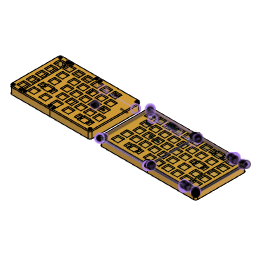
my-keyboard (Autodesk Fusion 360 design; units mm, degrees)
Autodesk Fusion 360 part; units mm, degrees
(part 1 of 2)
sketch "스케치1" plane through (0, 0, 0) normal (0, 0, 1) x (1, 0, 0)
  line L0 (0, 0) -> (143.11, 0)
  line L1 (143.11, 0) -> (143.11, 105.25)
  line L2 (143.11, 105.25) -> (0, 105.25)
  line L3 (0, 105.25) -> (0, 0)
  line L4 (0, 5) -> (143.11, 5) construction
  line L5 (0, 24.05) -> (143.11, 24.05) construction
  line L6 (0, 43.1) -> (143.11, 43.1) construction
  line L7 (0, 62.15) -> (143.11, 62.15) construction
  line L8 (0, 81.2) -> (143.11, 81.2) construction
  line L9 (2.525, 97.725) -> (16.525, 97.725)
  line L10 (16.525, 97.725) -> (16.525, 83.725)
  line L11 (16.525, 83.725) -> (2.525, 83.725)
  line L12 (2.525, 83.725) -> (2.525, 97.725)
  line L13 (7.2875, 64.675) -> (7.2875, 78.675)
  line L14 (7.2875, 78.675) -> (21.2875, 78.675)
  line L15 (21.2875, 78.675) -> (21.2875, 64.675)
  line L16 (21.2875, 64.675) -> (7.2875, 64.675)
  line L17 (21.575, 97.725) -> (35.575, 97.725)
  line L18 (21.575, 83.725) -> (21.575, 97.725)
  line L19 (35.575, 97.725) -> (35.575, 83.725)
  line L20 (35.575, 83.725) -> (21.575, 83.725)
  line L21 (40.625, 97.725) -> (54.625, 97.725)
  line L22 (40.625, 83.725) -> (40.625, 97.725)
  line L23 (54.625, 97.725) -> (54.625, 83.725)
  line L24 (54.625, 83.725) -> (40.625, 83.725)
  line L25 (59.675, 97.725) -> (73.675, 97.725)
  line L26 (59.675, 83.725) -> (59.675, 97.725)
  line L27 (73.675, 97.725) -> (73.675, 83.725)
  line L28 (73.675, 83.725) -> (59.675, 83.725)
  line L29 (78.725, 97.725) -> (92.725, 97.725)
  line L30 (78.725, 83.725) -> (78.725, 97.725)
  line L31 (92.725, 97.725) -> (92.725, 83.725)
  line L32 (92.725, 83.725) -> (78.725, 83.725)
  line L33 (97.775, 97.725) -> (111.775, 97.725)
  line L34 (97.775, 83.725) -> (97.775, 97.725)
  line L35 (111.775, 97.725) -> (111.775, 83.725)
  line L36 (111.775, 83.725) -> (97.775, 83.725)
  line L37 (31.1, 64.675) -> (31.1, 78.675)
  line L38 (31.1, 78.675) -> (45.1, 78.675)
  line L39 (45.1, 78.675) -> (45.1, 64.675)
  line L40 (45.1, 64.675) -> (31.1, 64.675)
  line L41 (64.15, 64.675) -> (50.15, 64.675)
  line L42 (64.15, 78.675) -> (64.15, 64.675)
  line L43 (50.15, 78.675) -> (64.15, 78.675)
  line L44 (50.15, 64.675) -> (50.15, 78.675)
  line L45 (83.2, 64.675) -> (69.2, 64.675)
  line L46 (83.2, 78.675) -> (83.2, 64.675)
  line L47 (69.2, 78.675) -> (83.2, 78.675)
  line L48 (69.2, 64.675) -> (69.2, 78.675)
  line L49 (102.25, 64.675) -> (88.25, 64.675)
  line L50 (102.25, 78.675) -> (102.25, 64.675)
  line L51 (88.25, 78.675) -> (102.25, 78.675)
  line L52 (88.25, 64.675) -> (88.25, 78.675)
  line L53 (121.3, 64.675) -> (107.3, 64.675)
  line L54 (121.3, 78.675) -> (121.3, 64.675)
  line L55 (107.3, 78.675) -> (121.3, 78.675)
  line L56 (107.3, 64.675) -> (107.3, 78.675)
  line L57 (23.66, 59.625) -> (23.66, 45.625)
  line L58 (9.66, 59.625) -> (23.66, 59.625)
  line L59 (9.66, 45.625) -> (9.66, 59.625)
  line L60 (23.66, 45.625) -> (9.66, 45.625)
  line L61 (35.845, 59.625) -> (49.845, 59.625)
  line L62 (35.845, 45.625) -> (35.845, 59.625)
  line L63 (49.845, 59.625) -> (49.845, 45.625)
  line L64 (49.845, 45.625) -> (35.845, 45.625)
  line L65 (54.895, 59.625) -> (68.895, 59.625)
  line L66 (54.895, 45.625) -> (54.895, 59.625)
  line L67 (68.895, 45.625) -> (54.895, 45.625)
  line L68 (68.895, 59.625) -> (68.895, 45.625)
  line L69 (73.945, 59.625) -> (87.945, 59.625)
  line L70 (73.945, 45.625) -> (73.945, 59.625)
  line L71 (87.945, 45.625) -> (73.945, 45.625)
  line L72 (87.945, 59.625) -> (87.945, 45.625)
  line L73 (92.995, 59.625) -> (106.995, 59.625)
  line L74 (92.995, 45.625) -> (92.995, 59.625)
  line L75 (106.995, 45.625) -> (92.995, 45.625)
  line L76 (106.995, 59.625) -> (106.995, 45.625)
  line L77 (112.045, 59.625) -> (126.045, 59.625)
  line L78 (112.045, 45.625) -> (112.045, 59.625)
  line L79 (126.045, 45.625) -> (112.045, 45.625)
  line L80 (126.045, 59.625) -> (126.045, 45.625)
  line L81 (14.4313, 40.575) -> (28.4313, 40.575)
  line L82 (28.4313, 26.575) -> (14.4313, 26.575)
  line L83 (45.3875, 40.575) -> (59.3875, 40.575)
  line L84 (45.3875, 26.575) -> (45.3875, 40.575)
  line L85 (59.3875, 26.575) -> (45.3875, 26.575)
  line L86 (59.3875, 40.575) -> (59.3875, 26.575)
  line L87 (64.4375, 40.575) -> (78.4375, 40.575)
  line L88 (78.4375, 40.575) -> (78.4375, 26.575)
  line L89 (78.4375, 26.575) -> (64.4375, 26.575)
  line L90 (64.4375, 26.575) -> (64.4375, 40.575)
  line L91 (83.4875, 40.575) -> (97.4875, 40.575)
  line L92 (97.4875, 40.575) -> (97.4875, 26.575)
  line L93 (97.4875, 26.575) -> (83.4875, 26.575)
  line L94 (83.4875, 26.575) -> (83.4875, 40.575)
  line L95 (102.5375, 40.575) -> (116.5375, 40.575)
  line L96 (116.5375, 40.575) -> (116.5375, 26.575)
  line L97 (116.5375, 26.575) -> (102.5375, 26.575)
  line L98 (102.5375, 26.575) -> (102.5375, 40.575)
  line L99 (121.5875, 40.575) -> (135.5875, 40.575)
  line L100 (135.5875, 40.575) -> (135.5875, 26.575)
  line L101 (135.5875, 26.575) -> (121.5875, 26.575)
  line L102 (121.5875, 26.575) -> (121.5875, 40.575)
  line L103 (18.9063, 7.525) -> (4.9062, 7.525)
  line L104 (18.9063, 21.525) -> (18.9063, 7.525)
  line L105 (4.9063, 7.525) -> (4.9063, 21.525)
  line L106 (4.9063, 21.525) -> (18.9063, 21.525)
  line L107 (28.7188, 21.525) -> (42.7188, 21.525)
  line L108 (28.7188, 7.525) -> (28.7188, 21.525)
  line L109 (42.7188, 21.525) -> (42.7188, 7.525)
  line L110 (42.7188, 7.525) -> (28.7188, 7.525)
  line L111 (52.5313, 21.525) -> (66.5313, 21.525)
  line L112 (52.5313, 7.525) -> (52.5313, 21.525)
  line L113 (66.5313, 21.525) -> (66.5313, 7.525)
  line L114 (66.5313, 7.525) -> (52.5313, 7.525)
  line L115 (76.3438, 21.525) -> (90.3438, 21.525)
  line L116 (76.3438, 7.525) -> (76.3438, 21.525)
  line L117 (90.3438, 21.525) -> (90.3438, 7.525)
  line L118 (90.3438, 7.525) -> (76.3438, 7.525)
  line L119 (6.1313, 39.075) -> (12.9313, 39.075)
  line L120 (12.9313, 28.075) -> (6.1313, 28.075)
  line L121 (6.1313, 28.075) -> (6.1313, 39.075)
  line L122 (29.9312, 39.075) -> (36.7313, 39.075)
  line L123 (36.7313, 39.075) -> (36.7313, 28.075)
  line L124 (36.7313, 28.075) -> (29.9313, 28.075)
  line L125 (12.9313, 39.075) -> (12.9313, 34.575)
  line L126 (12.9313, 32.575) -> (12.9313, 28.075)
  line L127 (14.4313, 26.575) -> (14.4313, 32.575)
  line L128 (14.4313, 34.575) -> (14.4313, 40.575)
  line L129 (28.4313, 40.575) -> (28.4312, 34.575)
  line L130 (28.4313, 32.575) -> (28.4313, 26.575)
  line L131 (29.9312, 28.075) -> (29.9312, 32.575)
  line L132 (29.9312, 34.575) -> (29.9312, 39.075)
  line L133 (29.9312, 32.575) -> (28.4312, 32.575)
  line L134 (14.4313, 32.575) -> (12.9313, 32.575)
  line L135 (12.9313, 34.575) -> (14.4313, 34.575)
  line L136 (28.4312, 34.575) -> (29.9313, 34.575)
  line L137 (131.9813, 9.025) -> (125.1813, 9.025)
  line L138 (123.6813, 15.525) -> (125.1813, 15.525)
  line L139 (123.6813, 21.525) -> (123.6813, 15.525)
  line L140 (131.9813, 20.025) -> (131.9813, 9.025)
  line L141 (125.1813, 13.525) -> (123.6813, 13.525)
  line L142 (101.3813, 9.025) -> (101.3813, 20.025)
  line L143 (108.1813, 20.025) -> (108.1813, 15.525)
  line L144 (101.3813, 20.025) -> (108.1813, 20.025)
  line L145 (123.6813, 7.525) -> (109.6813, 7.525)
  line L146 (109.6813, 15.525) -> (109.6813, 21.525)
  line L147 (125.1813, 15.525) -> (125.1813, 20.025)
  line L148 (108.1813, 15.525) -> (109.6813, 15.525)
  line L149 (125.1813, 9.025) -> (125.1813, 13.525)
  line L150 (125.1813, 20.025) -> (131.9813, 20.025)
  line L151 (109.6813, 13.525) -> (108.1813, 13.525)
  line L152 (109.6813, 7.525) -> (109.6813, 13.525)
  line L153 (108.1813, 13.525) -> (108.1813, 9.025)
  line L154 (108.1813, 9.025) -> (101.3813, 9.025)
  line L155 (123.6813, 13.525) -> (123.6813, 7.525)
  line L156 (109.6813, 21.525) -> (123.6813, 21.525)
  circle A0 centre (4, 4) radius 1.5
  circle A1 centre (4, 4) radius 3
  circle A2 centre (55.53, 4) radius 1.5
  circle A3 centre (55.53, 4) radius 3
  circle A4 centre (63.53, 4) radius 3
  circle A5 centre (63.53, 4) radius 1.5
  circle A6 centre (139.11, 4) radius 1.5
  circle A7 centre (139.11, 4) radius 3
  circle A8 centre (4, 101.25) radius 3
  circle A9 centre (4, 101.25) radius 1.5
  circle A10 centre (55.53, 101.25) radius 3
  circle A11 centre (55.53, 101.25) radius 1.5
  circle A12 centre (63.53, 101.25) radius 3
  circle A13 centre (63.53, 101.25) radius 1.5
  circle A14 centre (139.11, 101.25) radius 3
  circle A15 centre (139.11, 101.25) radius 1.5
  dimension "d1" = 105.25
  dimension "d2" = 143.11
  dimension "d5" = 5
  dimension "d8" = 0
  dimension "d9" = 19.05
  dimension "d10" = 14
  dimension "d11" = 14
  dimension "d14" = 2.525
  dimension "d15" = 2.525
  dimension "d20" = 14
  dimension "d21" = 14
  dimension "d22" = 2.525
  dimension "d23" = 7.2875
  dimension "d30" = 19.05
  dimension "d33" = 19.05
  dimension "d34" = 0
  dimension "d36" = 14
  dimension "d37" = 14
  dimension "d38" = 9.8125
  dimension "d44" = 19.05
  dimension "d45" = 0
  dimension "d46" = 14
  dimension "d47" = 14
  dimension "d48" = 9.66
  dimension "d49" = 2.525
  dimension "d50" = 14
  dimension "d51" = 14
  dimension "d52" = 12.185
  dimension "d55" = 19.05
  dimension "d56" = 0
  dimension "d57" = 14
  dimension "d58" = 14
  dimension "d59" = 2.525
  dimension "d60" = 14.4313
  dimension "d61" = 14
  dimension "d62" = 14
  dimension "d63" = 16.9563
  dimension "d66" = 19.05
  dimension "d67" = 0
  dimension "d68" = 14
  dimension "d69" = 14
  dimension "d70" = 4.9063
  dimension "d71" = 2.525
  dimension "d74" = 23.8125
  dimension "d75" = 0
  dimension "d76" = 6.8
  dimension "d77" = 11
  dimension "d78" = 1.5
  dimension "d80" = 4.5
  dimension "d81" = 6
  dimension "d82" = 14
  dimension "d83" = 14
  dimension "d84" = 6.8
  dimension "d85" = 11
  dimension "d86" = 1.5
  dimension "d87" = 4.5
  dimension "d88" = 6
  dimension "d89" = 19.3375
  dimension "d90" = 3
  dimension "d91" = 4
  dimension "d92" = 4
  dimension "d93" = 6
  dimension "d94" = 3
  dimension "d95" = 6
  dimension "d96" = 55.53
  dimension "d97" = 3
  dimension "d98" = 6
  dimension "d99" = 8
  dimension "d100" = 3
  dimension "d101" = 6
  dimension "d102" = 4
  dimension "d103" = 3
  dimension "d104" = 6
  dimension "d105" = 3
  dimension "d106" = 6
  dimension "d107" = 3
  dimension "d108" = 6
  dimension "d109" = 8
  dimension "d110" = 3
  dimension "d111" = 6
  dimension "d112" = 4
  dimension "d113" = 4
  dimension "d114" = 55.53
  dimension "d115" = 4
  constraint horizontal L0
  constraint vertical L1
  constraint horizontal L2
  constraint vertical L3
  constraint coincident L0.start L3.end
  constraint coincident L3 L4.start
  constraint perpendicular L3 L4
  constraint coincident L1 L4.end
  constraint horizontal L9
  constraint vertical L10
  constraint horizontal L11
  constraint vertical L12
  constraint horizontal L14
  constraint vertical L15
  constraint horizontal L16
  constraint vertical L13
  constraint horizontal L38
  constraint vertical L39
  constraint horizontal L40
  constraint vertical L37
  constraint horizontal L14.end L37.end
  constraint horizontal L58
  constraint vertical L57
  constraint horizontal L60
  constraint vertical L59
  constraint horizontal L61
  constraint vertical L63
  constraint horizontal L64
  constraint vertical L62
  constraint horizontal L57.start L61.start
  constraint horizontal L81
  constraint vertical L129
  constraint horizontal L82
  constraint vertical L127
  constraint horizontal L83
  constraint vertical L86
  constraint horizontal L85
  constraint vertical L84
  constraint horizontal L81.end L83.start
  constraint horizontal L106
  constraint vertical L104
  constraint horizontal L103
  constraint vertical L105
  constraint horizontal L119
  constraint vertical L125
  constraint horizontal L120
  constraint vertical L121
  constraint horizontal L135
  constraint horizontal L133
  constraint horizontal L122
  constraint vertical L123
  constraint horizontal L124
  constraint vertical L131
  constraint collinear L125 L126
  constraint coincident L127.end L133
  constraint collinear L127 L128
  constraint coincident L129.end L135
  constraint collinear L129 L130
  constraint collinear L131 L132
  constraint collinear L133 L134
  constraint collinear L135 L136
  constraint equal L119 L122
  constraint equal L121 L123
  constraint equal L125 L132
  constraint equal L135 L136
  constraint equal L125 L126
  constraint horizontal L156
  constraint vertical L139
  constraint horizontal L145
  constraint vertical L152
  constraint horizontal L144
  constraint vertical L143
  constraint horizontal L154
  constraint vertical L142
  constraint horizontal L148
  constraint horizontal L141
  constraint horizontal L150
  constraint vertical L140
  constraint horizontal L137
  constraint vertical L149
  constraint collinear L143 L153
  constraint coincident L151.start L141
  constraint collinear L146 L152
  constraint coincident L138.start L148
  constraint collinear L139 L155
  constraint collinear L147 L149
  constraint collinear L141 L151
  constraint collinear L138 L148
  constraint equal L144 L150
  constraint equal L140 L142
  constraint equal L143 L147
  constraint equal L138 L148
  constraint equal L143 L153
  constraint horizontal L115.end L146.end
  constraint concentric A0 A1
  constraint concentric A2 A3
  constraint horizontal A0.centre A2.centre
  constraint concentric A4 A5
  constraint horizontal A2.centre A4.centre
  constraint concentric A6 A7
  constraint horizontal A4.centre A6.centre
  constraint concentric A8 A9
  constraint concentric A10 A11
  constraint horizontal A10.centre A8.centre
  constraint concentric A12 A13
  constraint horizontal A12.centre A10.centre
  constraint concentric A14 A15
  constraint horizontal A12.centre A14.centre
  measures "d1" distance of L0.start L2.end
  measures "d2" distance of L1.end L2.end
  measures "d5" distance of L0.start L4.start
  measures "d10" distance of L9.start L9.end
  measures "d11" distance of L9.start L11.end
  measures "d14" vertical distance of L8.start L11.end
  measures "d15" horizontal distance of L8.start L11.end
  measures "d20" distance of L13.end L14.end
  measures "d21" distance of L13.end L13.start
  measures "d22" vertical distance of L7.start L13.start
  measures "d23" horizontal distance of L7.start L13.start
  measures "d30" distance of L4.start L5.start
  measures "d36" distance of L37.end L38.end
  measures "d37" distance of L37.start L37.end
  measures "d38" distance of L14.end L37.end
  measures "d46" distance of L58.start L57.start
  measures "d47" distance of L59.start L58.start
  measures "d48" horizontal distance of L7.start L58.start
  measures "d49" vertical distance of L7.start L58.start
  measures "d50" distance of L61.start L61.end
  measures "d51" distance of L62.start L61.start
  measures "d52" distance of L57.start L61.start
  measures "d57" distance of L81.start L81.end
  measures "d58" distance of L82.end L81.start
  measures "d59" vertical distance of L6.start L81.start
  measures "d60" horizontal distance of L6.start L81.start
  measures "d61" distance of L83.end L83.start
  measures "d62" distance of L84.start L83.start
  measures "d63" distance of L81.end L83.start
  measures "d68" distance of L104.start L105.end
  measures "d69" distance of L105.start L105.end
  measures "d70" horizontal distance of L5.start L105.end
  measures "d71" vertical distance of L5.start L105.end
  measures "d76" distance of L119.start L119.end
  measures "d77" distance of L119.start L120.end
  measures "d78" distance of L125.end L128.start
  measures "d80" distance of L119.end L125.end
  measures "d81" distance of L81.start L128.start
  measures "d82" distance of L139.start L146.end
  measures "d83" distance of L145.end L146.end
  measures "d84" distance of L142.end L143.start
  measures "d85" distance of L142.end L142.start
  measures "d86" distance of L146.start L143.end
  measures "d87" distance of L143.start L143.end
  measures "d88" distance of L146.start L146.end
  measures "d89" distance of L115.end L146.end
  measures "d90" diameter of A0
  measures "d91" horizontal distance of L0.start A0.centre
  measures "d92" vertical distance of L0.start A0.centre
  measures "d93" diameter of A1
  measures "d94" diameter of A2
  measures "d95" diameter of A3
  measures "d96" horizontal distance of L0.start A2.centre
  measures "d97" diameter of A5
  measures "d98" diameter of A4
  measures "d99" distance of A2.centre A4.centre
  measures "d100" diameter of A6
  measures "d101" diameter of A7
  measures "d102" horizontal distance of L0.end A6.centre
  measures "d103" diameter of A9
  measures "d104" diameter of A8
  measures "d105" diameter of A11
  measures "d106" diameter of A10
  measures "d107" diameter of A13
  measures "d108" diameter of A12
  measures "d109" distance of A12.centre A10.centre
  measures "d110" diameter of A15
  measures "d111" diameter of A14
  measures "d112" horizontal distance of L2.end A8.centre
  measures "d113" vertical distance of L2.end A8.centre
  measures "d114" horizontal distance of L2.end A10.centre
  measures "d115" horizontal distance of L1.end A14.centre
extrude "돌출1" add sketch "스케치1" along normal blind 3 contours L0 L1 L2 L3 | L9 L10 L11 L12 | L13 L14 L15 L16 | L17 L18 L19 L20 | L21 L22 L23 L24 | L25 L26 L27 L28 | L29 L30 L31 L32 | L33 L34 L35 L36 | L37 L38 L39 L40 | L41 L42 L43 L44 | L45 L46 L47 L48 | L49 L50 L51 L52 | L53 L54 L55 L56 | L57 L58 L59 L60 | L61 L62 L63 L64 | L65 L66 L67 L68 | L69 L70 L71 L72 | L73 L74 L75 L76 | L77 L78 L79 L80 | L81 L82 L119 L120 L121 L122 L123 L124 L125 L126 L127 L128 L129 L130 L131 L132 L133 L134 L135 L136 | L83 L84 L85 L86 | L87 L88 L89 L90 | L91 L92 L93 L94 | L95 L96 L97 L98 | L99 L100 L101 L102 | L103 L104 L105 L106 | L107 L108 L109 L110 | L111 L112 L113 L114 | L115 L116 L117 L118 | L137 L138 L139 L140 L141 L142 L143 L144 L145 L146 L147 L148 L149 L150 L151 L152 L153 L154 L155 L156 | A0 | A1 | A2 | A3 | A4 | A5 | A6 | A7 | A8 | A9 | A10 | A11 | A12 | A13 | A14 | A15 makes body 1
extrude "돌출2" cut sketch "스케치1" along normal through all contours L9 L10 L11 L12 | L13 L14 L15 L16 | L17 L18 L19 L20 | L21 L22 L23 L24 | L25 L26 L27 L28 | L29 L30 L31 L32 | L33 L34 L35 L36 | L37 L38 L39 L40 | L41 L42 L43 L44 | L45 L46 L47 L48 | L49 L50 L51 L52 | L53 L54 L55 L56 | L57 L58 L59 L60 | L61 L62 L63 L64 | L65 L66 L67 L68 | L69 L70 L71 L72 | L73 L74 L75 L76 | L77 L78 L79 L80 | L81 L82 L119 L120 L121 L122 L123 L124 L125 L126 L127 L128 L129 L130 L131 L132 L133 L134 L135 L136 | L83 L84 L85 L86 | L87 L88 L89 L90 | L91 L92 L93 L94 | L95 L96 L97 L98 | L99 L100 L101 L102 | L103 L104 L105 L106 | L107 L108 L109 L110 | L111 L112 L113 L114 | L115 L116 L117 L118 | L137 L138 L139 L140 L141 L142 L143 L144 L145 L146 L147 L148 L149 L150 L151 L152 L153 L154 L155 L156 | A0 | A2 | A5 | A6 | A9 | A11 | A13 | A15 bodies 1
sketch "스케치2" plane through (0, 0, 3) normal (0, 0, 1) x (-1, 0, 0)
  circle A0 centre (-55.53, -101.25) radius 1.5
  circle A1 centre (-63.53, -101.25) radius 1.5
  circle A2 centre (-139.11, -101.25) radius 1.5
  circle A3 centre (-139.11, -4) radius 1.5
  circle A4 centre (-63.53, -4) radius 1.5
  circle A5 centre (-55.53, -4) radius 1.5
  circle A6 centre (-4, -4) radius 1.5
  circle A7 centre (-4, -101.25) radius 3
  circle A8 centre (-55.53, -101.25) radius 3
  circle A9 centre (-63.53, -101.25) radius 3
  circle A10 centre (-139.11, -101.25) radius 3
  circle A11 centre (-139.11, -4) radius 3
  circle A12 centre (-63.53, -4) radius 3
  circle A13 centre (-55.53, -4) radius 3
  circle A14 centre (-4, -4) radius 3
  point P0 (-4, -101.25)
  point P1 (-55.53, -101.25)
  point P2 (-4, -4)
  dimension "d117" = 6
  dimension "d118" = 6
  dimension "d119" = 6
  dimension "d120" = 6
  dimension "d121" = 6
  dimension "d122" = 6
  dimension "d123" = 6
  dimension "d124" = 6
  constraint coincident P0 A7.centre
  constraint concentric A0 A8
  constraint concentric A1 A9
  constraint concentric A2 A10
  constraint concentric A3 A11
  constraint concentric A4 A12
  constraint concentric A5 A13
  constraint concentric A6 A14
  measures "d117" diameter of A7
  measures "d118" diameter of A8
  measures "d119" diameter of A9
  measures "d120" diameter of A10
  measures "d121" diameter of A11
  measures "d122" diameter of A12
  measures "d123" diameter of A13
  measures "d124" diameter of A14
extrude "돌출3" cut sketch "스케치2" against normal blind 1.5 bodies 1
copy_body "본체->구성요소1" bodies 1 removing the originals makes body 2 in component "left-switch"
sketch "스케치2 (2)" plane through (0, 0, 0) normal (0, 0, 1) x (1, 0, 0) in component "right-side-switch"
  line L0 (0, 0) -> (-24.05, 0)
  line L1 (-24.05, 0) -> (-24.05, 105.25)
  line L2 (-24.05, 105.25) -> (0, 105.25)
  line L3 (0, 105.25) -> (0, 0)
  line L4 (-16.525, 21.525) -> (-2.525, 21.525)
  line L5 (-2.525, 21.525) -> (-2.525, 7.525)
  line L6 (-2.525, 7.525) -> (-16.525, 7.525)
  line L7 (-16.525, 7.525) -> (-16.525, 21.525)
  line L8 (-16.525, 40.575) -> (-2.525, 40.575)
  line L9 (-2.525, 40.575) -> (-2.525, 26.575)
  line L10 (-2.525, 26.575) -> (-16.525, 26.575)
  line L11 (-16.525, 26.575) -> (-16.525, 40.575)
  line L12 (-16.525, 59.625) -> (-2.525, 59.625)
  line L13 (-2.525, 59.625) -> (-2.525, 45.625)
  line L14 (-2.525, 45.625) -> (-16.525, 45.625)
  line L15 (-16.525, 45.625) -> (-16.525, 59.625)
  line L16 (-16.525, 78.675) -> (-2.525, 78.675)
  line L17 (-2.525, 78.675) -> (-2.525, 64.675)
  line L18 (-2.525, 64.675) -> (-16.525, 64.675)
  line L19 (-16.525, 64.675) -> (-16.525, 78.675)
  line L20 (-16.525, 97.725) -> (-2.525, 97.725)
  line L21 (-2.525, 97.725) -> (-2.525, 83.725)
  line L22 (-2.525, 83.725) -> (-16.525, 83.725)
  line L23 (-16.525, 83.725) -> (-16.525, 97.725)
  circle A0 centre (-20.05, 101.25) radius 1.5
  circle A1 centre (-4, 101.25) radius 1.5
  circle A2 centre (-20.05, 4) radius 1.5
  circle A3 centre (-4, 4) radius 1.5
  point P0 (0, 105.25)
  dimension "d127" = 24.05
  dimension "d128" = 14
  dimension "d129" = 14
  dimension "d130" = 2.525
  dimension "d131" = 7.525
  dimension "d134" = 0
  dimension "d135" = 19.05
  dimension "d139" = 3
  dimension "d140" = 4
  dimension "d141" = 4
  dimension "d142" = 3
  dimension "d143" = 4
  dimension "d144" = 4
  dimension "d145" = 3
  dimension "d146" = 3
  dimension "d147" = 4
  dimension "d148" = 4
  dimension "d149" = 4
  dimension "d150" = 4
  constraint horizontal L0
  constraint vertical L1
  constraint horizontal L2
  constraint vertical L3
  constraint coincident L0.start L3.end
  constraint coincident P0 L2.end
  constraint horizontal L4
  constraint vertical L5
  constraint horizontal L6
  constraint vertical L7
  measures "d127" distance of L0.start L0.end
  measures "d128" distance of L4.start L4.end
  measures "d129" distance of L4.start L6.end
  measures "d130" horizontal distance of L0.start L5.end
  measures "d131" vertical distance of L0.start L5.end
  measures "d139" diameter of A0
  measures "d140" horizontal distance of L1.end A0.centre
  measures "d141" vertical distance of L1.end A0.centre
  measures "d142" diameter of A1
  measures "d143" horizontal distance of P0 A1.centre
  measures "d144" vertical distance of P0 A1.centre
  measures "d145" diameter of A2
  measures "d146" diameter of A3
  measures "d147" vertical distance of L0.end A2.centre
  measures "d148" horizontal distance of L0.end A2.centre
  measures "d149" horizontal distance of L0.start A3.centre
  measures "d150" vertical distance of L0.start A3.centre
extrude "돌출2'" add sketch "스케치2 (2)" along normal blind 3 separate body makes body 3 in component "right-side-switch"
sketch "스케치5" plane through (0, 0, 3) normal (0, 0, 1) x (-1, 0, 0) in component "right-side-switch"
  circle A0 centre (20.05, -101.25) radius 1.5
  circle A1 centre (4, -101.25) radius 1.5
  circle A2 centre (20.05, -4) radius 1.5
  circle A3 centre (4, -4) radius 1.5
  circle A4 centre (20.05, -101.25) radius 3
  circle A5 centre (4, -101.25) radius 3
  circle A6 centre (20.05, -4) radius 3
  circle A7 centre (4, -4) radius 3
  dimension "d159" = 6
  dimension "d160" = 6
  dimension "d161" = 6
  dimension "d162" = 6
  constraint concentric A0 A4
  constraint concentric A1 A5
  constraint concentric A2 A6
  constraint concentric A3 A7
  measures "d159" diameter of A4
  measures "d160" diameter of A5
  measures "d161" diameter of A6
  measures "d162" diameter of A7
extrude "돌출4" cut sketch "스케치5" against normal blind 1.5 bodies 3 in component "right-side-switch"
sketch "스케치1 (2)" plane through (0, 0, 0) normal (0, 0, 1) x (1, 0, 0) in component "left-body1"
  line L0 (0, 105.25) -> (-24.05, 105.25)
  line L1 (-24.05, 105.25) -> (-24.05, 0)
  line L2 (143.11, 105.25) -> (0, 105.25)
  line L3 (143.11, 0) -> (143.11, 105.25)
  line L4 (0, 0) -> (143.11, 0)
  line L5 (-24.05, 0) -> (0, 0)
  circle A0 centre (-20.05, 101.25) radius 1.5
  circle A1 centre (-4, 101.25) radius 1.5
  circle A2 centre (4, 101.25) radius 1.5
  circle A3 centre (-20.05, 4) radius 1.5
  circle A4 centre (-4, 4) radius 1.5
  circle A5 centre (4, 4) radius 1.5
  circle A6 centre (55.53, 101.25) radius 1.5
  circle A7 centre (55.53, 4) radius 1.5
  circle A8 centre (63.53, 4) radius 1.5
  circle A9 centre (63.53, 101.25) radius 1.5
  circle A10 centre (139.11, 4) radius 1.5
  circle A11 centre (139.11, 101.25) radius 1.5
  line L6 (-24.05, 105.25) -> (59.53, 105.25)
  line L7 (59.53, 105.25) -> (59.53, 0)
  line L8 (59.53, 0) -> (-24.05, 0)
  line L9 (-24.05, 0) -> (-24.05, 105.25)
  arc A12 (0, 4) -> (-7.873, 3) centre (-4, 4) ccw
  line L10 (51.657, 3) -> (7.873, 3)
  line L11 (-7.873, 3) -> (-16.177, 3)
  arc A13 (7.873, 3) -> (0, 4) centre (4, 4) ccw
  arc A14 (59.53, 4) -> (51.657, 3) centre (55.53, 4) ccw
  arc A15 (-16.177, 3) -> (-21.05, 7.873) centre (-20.05, 4) ccw
  arc A16 (51.657, 102.25) -> (59.53, 101.25) centre (55.53, 101.25) ccw
  arc A17 (0, 101.25) -> (7.873, 102.25) centre (4, 101.25) ccw
  arc A18 (-7.873, 102.25) -> (0, 101.25) centre (-4, 101.25) ccw
  arc A19 (-21.05, 97.377) -> (-16.177, 102.25) centre (-20.05, 101.25) ccw
  line L12 (-21.05, 97.377) -> (-21.05, 7.873)
  line L13 (-21.05, 5.118) -> (-21.05, 5)
  line L14 (-7.873, 102.25) -> (-16.177, 102.25)
  line L15 (51.657, 102.25) -> (7.873, 102.25)
  dimension "d166" = 4
  dimension "d167" = 8
  dimension "d168" = 8
  dimension "d169" = 8
  dimension "d170" = 8
  dimension "d171" = 3
  dimension "d172" = 8
  dimension "d173" = 8
  dimension "d174" = 8
  dimension "d175" = 8
  dimension "d176" = 3
  dimension "d178" = 3
  constraint horizontal L6
  constraint vertical L7
  constraint horizontal L8
  constraint vertical L9
  constraint coincident L4 L7.end
  constraint coincident L0.end L1.start
  constraint concentric A7 A14
  constraint horizontal L10
  constraint concentric A5 A13
  constraint concentric A4 A12
  constraint concentric A3 A15
  constraint coincident A12.end L10
  constraint collinear L10 L11
  constraint coincident L7 A14.start
  constraint concentric A0 A19
  constraint concentric A1 A18
  constraint concentric A2 A17
  constraint concentric A6 A16
  constraint horizontal L15
  constraint coincident L7 A16.end
  constraint coincident A18.start L15
  constraint vertical L12
  constraint coincident A3 L13.start
  constraint collinear L12 L13
  constraint parallel L6 L14
  measures "d166" horizontal distance of A7.centre L7.end
  measures "d167" diameter of A14
  measures "d168" diameter of A13
  measures "d169" diameter of A12
  measures "d170" diameter of A15
  measures "d171" vertical distance of L7.end L10.start
  measures "d172" diameter of A19
  measures "d173" diameter of A18
  measures "d174" diameter of A17
  measures "d175" diameter of A16
  measures "d176" vertical distance of L6.end A16.start
  measures "d178" horizontal distance of L0.end A19.start
extrude "돌출1'" add sketch "스케치1 (2)" against normal blind 13 separate body contours L0 L1 L2 L4 L5 L6 L7 L8 L9 A12 L10 L11 A13 A14 A15 A16 A17 A18 A19 L12 L14 L15 | L7 A12 L10 L11 A13 A14 A15 A16 A17 A18 A19 L12 L14 L15 | A0 | A1 | A2 | A3 | A4 | A5 | A6 | A7 makes body 4 in component "left-body1"
extrude "돌출2''" cut sketch "스케치1 (2)" against normal blind 12 contours L7 A12 L10 L11 A13 A14 A15 A16 A17 A18 A19 L12 L14 L15 bodies 4 in component "left-body1"
extrude "돌출3'" cut sketch "스케치1 (2)" against normal blind 8 contours A0 | A1 | A2 | A3 | A4 | A5 | A6 | A7 bodies 4 in component "left-body1"
sketch "스케치2 (3)" plane through (0, 0, 0) normal (0, 0, 1) x (1, 0, 0) in component "left-body2"
  line L0 (59.53, 105.25) -> (59.53, 0)
  line L1 (143.11, 105.25) -> (0, 105.25)
  line L2 (143.11, 0) -> (143.11, 105.25)
  line L3 (0, 0) -> (143.11, 0)
  circle A0 centre (63.53, 4) radius 1.5
  circle A1 centre (139.11, 4) radius 1.5
  circle A2 centre (139.11, 101.25) radius 1.5
  circle A3 centre (63.53, 101.25) radius 1.5
  line L4 (67.403, 102.25) -> (135.237, 102.25)
  line L5 (140.11, 99) -> (140.11, 7.873)
  line L6 (135.237, 3) -> (67.403, 3)
  arc A4 (67.403, 3) -> (59.53, 4) centre (63.53, 4) ccw
  arc A5 (140.11, 7.873) -> (135.237, 3) centre (139.11, 4) ccw
  arc A6 (135.237, 102.25) -> (140.11, 97.377) centre (139.11, 101.25) ccw
  arc A7 (59.53, 101.25) -> (67.403, 102.25) centre (63.53, 101.25) ccw
  circle A8 centre (63.53, 101.25) radius 1.5
  circle A9 centre (139.11, 101.25) radius 1.5
  circle A10 centre (139.11, 4) radius 1.5
  circle A11 centre (139.11, 4) radius 1.5
  circle A12 centre (139.11, 4) radius 1.5
  circle A13 centre (63.53, 4) radius 1.5
  circle A14 centre (63.53, 4) radius 1.5
  point P0 (63.53, 4)
  point P1 (59.53, 0)
  dimension "d185" = 8
  dimension "d186" = 8
  dimension "d187" = 8
  dimension "d188" = 8
  dimension "d189" = 3
  dimension "d190" = 3
  dimension "d191" = 3
  dimension "d192" = 3
  dimension "d193" = 3
  dimension "d194" = 3
  dimension "d195" = 3
  constraint concentric A3 A7
  constraint concentric A2 A6
  constraint coincident P0 A0.centre
  constraint concentric A1 A5
  constraint horizontal L4
  constraint parallel L2 L5
  constraint horizontal L6
  constraint coincident L0 A4.end
  constraint coincident L5 A6.end
  constraint coincident L0 A7.start
  constraint concentric A3 A8
  constraint concentric A2 A9
  constraint concentric A1 A10
  constraint concentric A10 A11
  constraint concentric A1 A12
  constraint concentric A4 A14
  measures "d185" diameter of A7
  measures "d186" diameter of A6
  measures "d187" diameter of A4
  measures "d188" diameter of A5
  measures "d189" vertical distance of L6.end P1
  measures "d190" horizontal distance of L2.start L5.end
  measures "d191" vertical distance of L1.start L4.end
  measures "d192" diameter of A8
  measures "d193" diameter of A9
  measures "d194" diameter of A12
  measures "d195" diameter of A14
extrude "돌출1''" add sketch "스케치2 (3)" against normal blind 13 separate body contours L0 L1 L2 L3 L4 L5 L6 A4 A5 A6 A7 | L0 L4 L5 L6 A4 A5 A6 A7 | A0 A13 A14 | A1 A10 A11 A12 | A2 A9 | A3 A8 makes body 5 in component "left-body2"
extrude "돌출2'''" cut sketch "스케치2 (3)" against normal blind 12 contours L0 L4 L5 L6 A4 A5 A6 A7 bodies 5 in component "left-body2"
extrude "돌출3''" cut sketch "스케치1 (2)" against normal blind 8 contours A8 | A9 | A10 | A11 bodies 5 in component "left-body2"
sketch "스케치4" plane through (0, 105.25, 0) normal (0, 1, 0) x (-1, 0, 0) in component "left-body2"
  line L0 (-67.403, -12) -> (-135.237, -12) construction
  circle A0 centre (-129.837, -9) radius 3.2
  line L1 (-99.287, -10.5) -> (-93.487, -10.5)
  arc A1 (-93.487, -10.5) -> (-93.487, -7.1) centre (-93.487, -8.8) ccw
  line L2 (-93.487, -7.1) -> (-99.287, -7.1)
  arc A2 (-99.287, -7.1) -> (-99.287, -10.5) centre (-99.287, -8.8) ccw
  line L3 (-99.287, -8.8) -> (-93.487, -8.8) construction
  line L4 (-99.287, -12.5) -> (-93.487, -12.5)
  arc A3 (-93.487, -12.5) -> (-93.487, -5.1) centre (-93.487, -8.8) ccw
  line L5 (-93.487, -5.1) -> (-99.287, -5.1)
  arc A4 (-99.287, -5.1) -> (-99.287, -12.5) centre (-99.287, -8.8) ccw
  line L6 (-99.287, -8.8) -> (-93.487, -8.8) construction
  dimension "d202" = 6.4
  dimension "d203" = 3
  dimension "d204" = 5.4
  dimension "d205" = 3.4
  dimension "d206" = 5.8
  dimension "d207" = 1.5
  dimension "d208" = 7.4
  dimension "d236" = 35.95
  constraint tangent L1 A1
  constraint tangent A1 L2
  constraint parallel L1 L2
  constraint tangent L2 A2
  constraint tangent L1 A2
  constraint parallel L0 L3
  constraint tangent L4 A3
  constraint tangent A3 L5
  constraint parallel L4 L5
  constraint tangent L5 A4
  constraint tangent L4 A4
  constraint coincident A1.centre L3.end
  constraint parallel L3 L6
  constraint coincident A2.centre L3.start
  measures "d202" diameter of A0
  measures "d203" vertical distance of L0.end A0.centre
  measures "d204" horizontal distance of L0.end A0.centre
  measures "d205" diameter of A1
  measures "d206" distance of A2.centre A1.centre
  measures "d207" vertical distance of L0.end L1.start
  measures "d208" diameter of A3
  measures "d236" horizontal distance of L0.end L1.start
sketch "스케치5 (2)" plane through (0, 0, -12) normal (0, 0, 1) x (-1, 0, 0) in component "left-body2"
  line L0 (-87.237, -65.65) -> (-105.237, -65.65)
  line L1 (-105.237, -65.65) -> (-105.237, -66.65)
  line L2 (-105.237, -66.65) -> (-87.237, -66.65)
  line L3 (-87.237, -66.65) -> (-87.237, -65.65)
  line L4 (-121.237, -86.25) -> (-133.237, -86.25)
  line L5 (-133.237, -86.25) -> (-133.237, -87.25)
  line L6 (-133.237, -87.25) -> (-121.237, -87.25)
  line L7 (-121.237, -87.25) -> (-121.237, -86.25)
  line L8 (-67.403, -102.25) -> (-135.237, -102.25)
  point P0 (-135.237, -102.25)
  dimension "d216" = 18
  dimension "d217" = 1
  dimension "d218" = 2
  dimension "d219" = 12
  dimension "d220" = 1
  dimension "d221" = 15
  dimension "d222" = 30
  dimension "d223" = 35.6
  constraint horizontal L0
  constraint vertical L1
  constraint horizontal L2
  constraint vertical L3
  constraint horizontal L4
  constraint vertical L5
  constraint horizontal L6
  constraint vertical L7
  measures "d216" distance of L0.start L0.end
  measures "d217" distance of L0.start L2.end
  measures "d218" horizontal distance of L5.end P0
  measures "d219" distance of L4.start L4.end
  measures "d220" distance of L4.start L6.end
  measures "d221" vertical distance of L5.end P0
  measures "d222" horizontal distance of L1.end P0
  measures "d223" vertical distance of L1.end P0
extrude "돌출4'" add sketch "스케치5 (2)" along normal blind 2 bodies 5 in component "left-body2"
extrude "돌출5" cut sketch "스케치4" against normal blind 3 contours A0 | L1 A1 L2 A2 bodies 5 in component "left-body2"
extrude "돌출6" cut sketch "스케치4" against normal blind 2 contours L4 A3 L5 A4 bodies 5 in component "left-body2"
sketch "스케치6" plane through (87.237, 0, 0) normal (-1, 0, 0) x (0, -1, 0) in component "left-body2"
  line L0 (-66.65, -12) -> (-66.65, -10)
  line L1 (-66.65, -10) -> (-65.65, -10)
  line L2 (-65.65, -10) -> (-65.65, -8.5)
  line L3 (-65.65, -8.5) -> (-67.0488, -10)
  line L4 (-67.0488, -10) -> (-65.65, -10)
  dimension "d230" = 1.5
  dimension "d231" = 47
  constraint coincident L1.end L2.start
  constraint perpendicular L1 L2
  constraint perpendicular L2 L4
  measures "d230" distance of L1.end L2.end
  measures "d231" angle of L3 L4
extrude "돌출7" add sketch "스케치6" against normal blind 18 bodies 5 in component "left-body2"
fillet "모깎기1" radius 0.2 1 edges at (96.237, 65.65, -8.5) on bodies 5 in component "left-body2"
sketch "스케치6 (2)" plane through (0, 0, 0) normal (0, 0, 1) x (1, 0, 0) in component "right-side-switch"